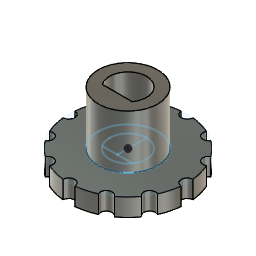
turning knob (Autodesk Fusion 360 design; units mm, degrees)
Autodesk Fusion 360 part; units mm, degrees
sketch "Skizze1" plane through (0, 0, 0) normal (0, 0, 1) x (1, 0, 0)
  circle A0 centre (0, 0) radius 10
  constraint coincident A0.centre origin
extrude "Extrusion1" add sketch "Skizze1" along normal blind 3
sketch "Skizze2" plane through (0, 0, 3) normal (0, 0, 1) x (-1, 0, 0)
  circle A0 centre (0, 0) radius 10
  circle A1 centre (0, 0) radius 3.1015
  circle A2 centre (0, 0) radius 5
  line L0 (0, -3.1015) -> (0, 1.7)
  line L1 (0, 1.7) -> (0, 1.8)
  line L2 (0, 1.8) -> (-2.5258, 1.8)
  line L3 (0, 1.8) -> (2.5258, 1.8)
  constraint coincident A0.centre A1.centre
  constraint coincident A1 L0.start
  constraint vertical L0
  constraint coincident A1 L2.end
  constraint perpendicular L1 L2
  constraint coincident A1 L3.end
  constraint perpendicular L1 L3
cylinder "Grundkörper Zylinder1" cut diameter 2 height -3 placed x (0, 1, 0) y (1, 0, 0) z (0, 0, -1) at (0, -10, 0)
pattern_circular "C-Anordnung1" count 12 over 360 about axis through (0, 0, 0) along (0, 0, 1) of 1 faces at (0.9952, -9.9019, 2)
sketch "Skizze4" plane through (0, 0, 3) normal (0, 0, 1) x (-1, 0, 0)
extrude "Extrusion5" add sketch "Skizze2" along normal blind 9 contours A1 L2 L3 | A2
